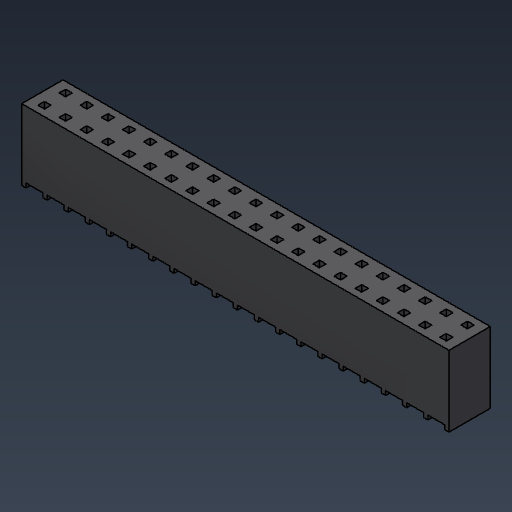
# Autodesk Inventor part: SSW-120-01-F-D_terminal
Saved by Autodesk Inventor 2023.1 (Build 271208000, 208)
## iProperties
Category: PARTsolutions
Company: SAMTEC
Created: 2015-08-09
Part Number: SSW-120-01-F-D_terminal
Catalog Web Link: www.cadenas.de
Description: SSW Series Terminal-SSW Series - (2,54 mm) .100" Surface Mount Terminal & Through-Hole .025" Square Post Socket
Vendor: SAMTEC
Document SubType Name: Modeling
Designer: PARTuser1
Manufacturer: SAMTEC
Mass: 1.8617 g
Surface Area: 24.8346 cm^2
Volume: 1.8617 cm^3
Density: 1 g/cm^3
Material: Allgemein
Appearance: PSOLRGB-175-175-175
PSOL_IDENT_0: {$CADENAS_DATA\23d-libs\samtec\modelling\ssw\parts\ssw_terminal.prj},256 {VTYP=3D},{NB=SSW-120-01-F-
PSOL_IDENT_1: D_terminal},{LINA=SSW-120-01-F-D_terminal},{NN=SSW Series Terminal},{DATE=20.05.2015 07:57:00},{GEOM
PSOL_IDENT_2: DATE=20.05.2015 07:56:00},{VERSION=},{LINEID=10},{LINESUBID=-1},{WBVAR=POS,LS,PLOPT,ROW,TOPT,POLOPT,
PSOL_IDENT_3: NOPT,LLOPT,POPT,KOPT,TROPT}  {NB=SSW-120-01-F-D_terminal},{LINA=SSW-120-01-F-D_terminal},{KT=DUMMY},
PSOL_IDENT_4: {PN=SSW-120-01-F-D},{SERIES=SSW},{POS=20},{POSATOF=20},{LS=01},{LSALG= '01','-01','02','-02','03','-
PSOL_IDENT_5: 03','04','-04','06','-06','21','-21','22','-22','23','-23','24','-24' },{PLOPT=F},{PLOPTALG= 'G','-G
PSOL_IDENT_6: - Gold, 20micro\" Au / 50micro\" Ni Min on Contact, 3micro\" Au / 50micro\" Ni Min on Tail','S','-S
PSOL_IDENT_7: - Selective, 30micro\" Au / 50micro\" Ni Min on Contact, Matte Tin Tail','H','-H - Heavy Gold 30mic
PSOL_IDENT_8: ro\" Au / 50micro\" Ni Min on Contact, 3micro\" Au / 50micro\" Ni Min on Tail' ,'F','-F - Flash Sele
PSOL_IDENT_9: ctive, 3micro\" Au / 50micro\" Ni Min on Contact, Matte Tin Tail','STL','-STL - Selective, 30micro\"
PSOL_IDENT_10: Au / 50micro\" Ni Min on Contact Area, Tin/Lead (90/10 +/-5%) Tail','SM','-SM - Selective, 30micro\
PSOL_IDENT_11: " Au / 50micro\" Ni Min on Contact, Matte Tin Tail','FM','-FM - Flash Selective, 3micro\" Au / 50mic
PSOL_IDENT_12: ro\" Ni Min on Contact, Matte Tin Tail','L','-L - Light Selective, 10micro\" Au / 50micro\" Ni Min o
PSOL_IDENT_13: n Contact Area, Matte Tin Tail','T','-T - Matte Tin Contact and Tail','E','-E - 50micro\" Extra Heav
PSOL_IDENT_14: y Gold in Contact Area, 3micro\" Gold on Tail','TL','-TL - Tin/Lead (90/10 ± 5%) Contact and Tail','
PSOL_IDENT_15: TM','-TM - Matte Tin Contact and Tail' },{ROW=D},{ROWALG= 'S','-S - Single','D','-D - Double','T','-
PSOL_IDENT_16: T - Triple', 'P','-P - Single Notched','Q','-Q - Triple with only Outer 2 Rows Filled' },{TOPT=},{TO
PSOL_IDENT_17: PTALG= '','Straight' },{TOPTPN=},{POLOPT=},{POLOPTALG= '','Not Selected','001','001','002','002','00
PSOL_IDENT_18: 3','003','004','004','005','005','006','006','007','007','008','008','009','009','010','010','011','
PSOL_IDENT_19: 011','012','012','013','013','014','014','015','015','016','016','017','017','018','018','019','019'
PSOL_IDENT_20: ,'020','020','021','021','022','022','023','023','024','024','025','025','026','026','027','027','02
PSOL_IDENT_21: 8','028','029','029','030','030','031','031','032','032','033','033','034','034','035','035','036','
PSOL_IDENT_22: 036','037','037','038','038','039','039','040','040' },{POLOPTMAX=480},{POLOPTMAX2='001','001','002'
PSOL_IDENT_23: ,'002','003','003','004','004','005','005','006','006','007','007','008','008','009','009','010','01
PSOL_IDENT_24: 0','011','011','012','012','013','013','014','014','015','015','016','016','017','017','018','018','
PSOL_IDENT_25: 019','019','020','020','021','021','022','022','023','023','024','024','025','025','026','026','027'
PSOL_IDENT_26: ,'027','028','028','029','029','030','030','031','031','032','032','033','033','034','034','035','03
PSOL_IDENT_27: 5','036','036','037','037','038','038','039','039','040','040'},{POLARIZE='001','001','002','002','0
PSOL_IDENT_28: 03','003','004','004','005','005','006','006','007','007','008','008','009','009','010','010','011','
PSOL_IDENT_29: 011','012','012','013','013','014','014','015','015','016','016','017','017','018','018','019','019'
PSOL_IDENT_30: ,'020','020','021','021','022','022','023','023','024','024','025','025','026','026','027','027','02
PSOL_IDENT_31: 8','028','029','029','030','030','031','031','032','032','033','033','034','034','035','035','036','
PSOL_IDENT_32: 036','037','037','038','038','039','039','040','040','041','041','042','042','043','043','044','044'
PSOL_IDENT_33: ,'045','045','046','046','047','047','048','048','049','049','050','050','051','051','052','052','05
PSOL_IDENT_34: 3','053','054','054','055','055','056','056','057','057','058','058','059','059','060','060','061','
PSOL_IDENT_35: 061','062','062','063','063','064','064','065','065','066','066','067','067','068','068','069','069'
PSOL_IDENT_36: ,'070','070','071','071','072','072','073','073','074','074','075','075','076','076','077','077','07
PSOL_IDENT_37: 8','078','079','079','080','080','081','081','082','082','083','083','084','084','085','085','086','
PSOL_IDENT_38: 086','087','087','088','088','089','089','090','090','091','091','092','092','093','093','094','094'
PSOL_IDENT_39: ,'095','095','096','096','097','097','098','098','099','099','100','100','101','101','102','102','10
PSOL_IDENT_40: 3','103','104','104','105','105','106','106','107','107','108','108','109','109','110','110','111','
PSOL_IDENT_41: 111','112','112','113','113','114','114','115','115','116','116','117','117','118','118','119','119'
PSOL_IDENT_42: ,'120','120','121','121','122','122','123','123','124','124','125','125','126','126','127','127','12
PSOL_IDENT_43: 8','128','129','129','130','130','131','131','132','132','133','133','134','134','135','135','136','
PSOL_IDENT_44: 136','137','137','138','138','139','139','140','140','141','141','142','142','143','143','144','144'
PSOL_IDENT_45: ,'145','145','146','146','147','147','148','148','149','149','150','150'},{POLOPTPN=},{NOPT=},{NOPTA
PSOL_IDENT_46: LG= '','Not Selected','N','-N - Notch' },{NOPTPN=},{LLOPT=},{LLOPTALG= '','Not Selected','LL','-LL -
PSOL_IDENT_47: Locking Lead' },{LLOPTPN=},{POPT=},{POPTALG= '','Not Available' },{POPTPN=},{KOPT=},{KOPTALG= '','N
PSOL_IDENT_48: ot Available' },{KOPTPN=},{TROPT=},{TROPTALG= '','Not Available' },{TROPTPN=},{B=0.104},{C=0.000},{R=
PSOL_IDENT_49: 2.020},{APOPT=0.81250},{CPOPT=0.89750},{SKOPT=0.88200},{OEN=2},{POSX=1.01500},{POSY=0.01500},{POLOPT
PSOL_IDENT_50: ATOF=0},{POLMOVE=2}
NN: SSW Series Terminal
NT: SSW Series - (2,54 mm) .100" Surface Mount Terminal & Through-Hole .025" Square Post Socket
NB: SSW-120-01-F-D_terminal
NBSYN: $PN._terminal
LINA: SSW-120-01-F-D_terminal
SERIES: SSW
POS: -20
LS: -01
PLOPT: -F - Flash Selective, 3micro" Au / 50micro" Ni Min on Contact, Matte Tin Tail
ROW: -D - Double
TOPT: Straight
POLOPT: Not Selected
NOPT: Not Selected
LLOPT: Not Selected
POPT: Not Available
KOPT: Not Available
TROPT: Not Available
SUPPLIER: SAMTEC
ARTICLENO: SSW-120-01-F-D_terminal
BOMINFO: SSW-120-01-F-D_terminal
CREATOR: CADENAS GmbH
Title: SSW-120-01-F-D_terminal
Author: Cadenas PARTsolutions
Comments: SSW Series - (2,54 mm) .100" Surface Mount Terminal & Through-Hole .025" Square Post Socket
Autodesk Inventor part; units mm, degrees
sketch "Sketch_1" plane through (0, 0, 0) normal (0, 1, 0) x (-1, 0, 0)
  line L0 (25.654, -2.4765) -> (25.654, 2.4765)
  line L1 (25.654, 2.4765) -> (-25.654, 2.4765)
  line L2 (-25.654, 2.4765) -> (-25.654, -2.4765)
  line L3 (-25.654, -2.4765) -> (25.654, -2.4765)
  line L4 (-23.7363, 0.8763) -> (-23.7363, 1.6637)
  line L5 (-23.7363, 1.6637) -> (-24.5237, 1.6637)
  line L6 (-24.5237, 1.6637) -> (-24.5237, 0.8763)
  line L7 (-24.5237, 0.8763) -> (-23.7363, 0.8763)
  line L8 (-23.7363, -1.6637) -> (-23.7363, -0.8763)
  line L9 (-23.7363, -0.8763) -> (-24.5237, -0.8763)
  line L10 (-24.5237, -0.8763) -> (-24.5237, -1.6637)
  line L11 (-24.5237, -1.6637) -> (-23.7363, -1.6637)
  line L12 (-21.1963, 0.8763) -> (-21.1963, 1.6637)
  line L13 (-21.1963, 1.6637) -> (-21.9837, 1.6637)
  line L14 (-21.9837, 1.6637) -> (-21.9837, 0.8763)
  line L15 (-21.9837, 0.8763) -> (-21.1963, 0.8763)
  line L16 (-21.1963, -1.6637) -> (-21.1963, -0.8763)
  line L17 (-21.1963, -0.8763) -> (-21.9837, -0.8763)
  line L18 (-21.9837, -0.8763) -> (-21.9837, -1.6637)
  line L19 (-21.9837, -1.6637) -> (-21.1963, -1.6637)
  line L20 (-18.6563, 0.8763) -> (-18.6563, 1.6637)
  line L21 (-18.6563, 1.6637) -> (-19.4437, 1.6637)
  line L22 (-19.4437, 1.6637) -> (-19.4437, 0.8763)
  line L23 (-19.4437, 0.8763) -> (-18.6563, 0.8763)
  line L24 (-18.6563, -1.6637) -> (-18.6563, -0.8763)
  line L25 (-18.6563, -0.8763) -> (-19.4437, -0.8763)
  line L26 (-19.4437, -0.8763) -> (-19.4437, -1.6637)
  line L27 (-19.4437, -1.6637) -> (-18.6563, -1.6637)
  line L28 (-16.1163, 0.8763) -> (-16.1163, 1.6637)
  line L29 (-16.1163, 1.6637) -> (-16.9037, 1.6637)
  line L30 (-16.9037, 1.6637) -> (-16.9037, 0.8763)
  line L31 (-16.9037, 0.8763) -> (-16.1163, 0.8763)
  line L32 (-16.1163, -1.6637) -> (-16.1163, -0.8763)
  line L33 (-16.1163, -0.8763) -> (-16.9037, -0.8763)
  line L34 (-16.9037, -0.8763) -> (-16.9037, -1.6637)
  line L35 (-16.9037, -1.6637) -> (-16.1163, -1.6637)
  line L36 (-13.5763, 0.8763) -> (-13.5763, 1.6637)
  line L37 (-13.5763, 1.6637) -> (-14.3637, 1.6637)
  line L38 (-14.3637, 1.6637) -> (-14.3637, 0.8763)
  line L39 (-14.3637, 0.8763) -> (-13.5763, 0.8763)
  line L40 (-13.5763, -1.6637) -> (-13.5763, -0.8763)
  line L41 (-13.5763, -0.8763) -> (-14.3637, -0.8763)
  line L42 (-14.3637, -0.8763) -> (-14.3637, -1.6637)
  line L43 (-14.3637, -1.6637) -> (-13.5763, -1.6637)
  line L44 (-11.0363, 0.8763) -> (-11.0363, 1.6637)
  line L45 (-11.0363, 1.6637) -> (-11.8237, 1.6637)
  line L46 (-11.8237, 1.6637) -> (-11.8237, 0.8763)
  line L47 (-11.8237, 0.8763) -> (-11.0363, 0.8763)
  line L48 (-11.0363, -1.6637) -> (-11.0363, -0.8763)
  line L49 (-11.0363, -0.8763) -> (-11.8237, -0.8763)
  line L50 (-11.8237, -0.8763) -> (-11.8237, -1.6637)
  line L51 (-11.8237, -1.6637) -> (-11.0363, -1.6637)
  line L52 (-8.4963, 0.8763) -> (-8.4963, 1.6637)
  line L53 (-8.4963, 1.6637) -> (-9.2837, 1.6637)
  line L54 (-9.2837, 1.6637) -> (-9.2837, 0.8763)
  line L55 (-9.2837, 0.8763) -> (-8.4963, 0.8763)
  line L56 (-8.4963, -1.6637) -> (-8.4963, -0.8763)
  line L57 (-8.4963, -0.8763) -> (-9.2837, -0.8763)
  line L58 (-9.2837, -0.8763) -> (-9.2837, -1.6637)
  line L59 (-9.2837, -1.6637) -> (-8.4963, -1.6637)
  line L60 (-5.9563, 0.8763) -> (-5.9563, 1.6637)
  line L61 (-5.9563, 1.6637) -> (-6.7437, 1.6637)
  line L62 (-6.7437, 1.6637) -> (-6.7437, 0.8763)
  line L63 (-6.7437, 0.8763) -> (-5.9563, 0.8763)
  line L64 (-5.9563, -1.6637) -> (-5.9563, -0.8763)
  line L65 (-5.9563, -0.8763) -> (-6.7437, -0.8763)
  line L66 (-6.7437, -0.8763) -> (-6.7437, -1.6637)
  line L67 (-6.7437, -1.6637) -> (-5.9563, -1.6637)
  line L68 (-3.4163, 0.8763) -> (-3.4163, 1.6637)
  line L69 (-3.4163, 1.6637) -> (-4.2037, 1.6637)
  line L70 (-4.2037, 1.6637) -> (-4.2037, 0.8763)
  line L71 (-4.2037, 0.8763) -> (-3.4163, 0.8763)
  line L72 (-3.4163, -1.6637) -> (-3.4163, -0.8763)
  line L73 (-3.4163, -0.8763) -> (-4.2037, -0.8763)
  line L74 (-4.2037, -0.8763) -> (-4.2037, -1.6637)
  line L75 (-4.2037, -1.6637) -> (-3.4163, -1.6637)
  line L76 (-0.8763, 0.8763) -> (-0.8763, 1.6637)
  line L77 (-0.8763, 1.6637) -> (-1.6637, 1.6637)
  line L78 (-1.6637, 1.6637) -> (-1.6637, 0.8763)
  line L79 (-1.6637, 0.8763) -> (-0.8763, 0.8763)
  line L80 (-0.8763, -1.6637) -> (-0.8763, -0.8763)
  line L81 (-0.8763, -0.8763) -> (-1.6637, -0.8763)
  line L82 (-1.6637, -0.8763) -> (-1.6637, -1.6637)
  line L83 (-1.6637, -1.6637) -> (-0.8763, -1.6637)
  line L84 (1.6637, 0.8763) -> (1.6637, 1.6637)
  line L85 (1.6637, 1.6637) -> (0.8763, 1.6637)
  line L86 (0.8763, 1.6637) -> (0.8763, 0.8763)
  line L87 (0.8763, 0.8763) -> (1.6637, 0.8763)
  line L88 (1.6637, -1.6637) -> (1.6637, -0.8763)
  line L89 (1.6637, -0.8763) -> (0.8763, -0.8763)
  line L90 (0.8763, -0.8763) -> (0.8763, -1.6637)
  line L91 (0.8763, -1.6637) -> (1.6637, -1.6637)
  line L92 (4.2037, 0.8763) -> (4.2037, 1.6637)
  line L93 (4.2037, 1.6637) -> (3.4163, 1.6637)
  line L94 (3.4163, 1.6637) -> (3.4163, 0.8763)
  line L95 (3.4163, 0.8763) -> (4.2037, 0.8763)
  line L96 (4.2037, -1.6637) -> (4.2037, -0.8763)
  line L97 (4.2037, -0.8763) -> (3.4163, -0.8763)
  line L98 (3.4163, -0.8763) -> (3.4163, -1.6637)
  line L99 (3.4163, -1.6637) -> (4.2037, -1.6637)
  line L100 (6.7437, 0.8763) -> (6.7437, 1.6637)
  line L101 (6.7437, 1.6637) -> (5.9563, 1.6637)
  line L102 (5.9563, 1.6637) -> (5.9563, 0.8763)
  line L103 (5.9563, 0.8763) -> (6.7437, 0.8763)
  line L104 (6.7437, -1.6637) -> (6.7437, -0.8763)
  line L105 (6.7437, -0.8763) -> (5.9563, -0.8763)
  line L106 (5.9563, -0.8763) -> (5.9563, -1.6637)
  line L107 (5.9563, -1.6637) -> (6.7437, -1.6637)
  line L108 (9.2837, 0.8763) -> (9.2837, 1.6637)
  line L109 (9.2837, 1.6637) -> (8.4963, 1.6637)
  line L110 (8.4963, 1.6637) -> (8.4963, 0.8763)
  line L111 (8.4963, 0.8763) -> (9.2837, 0.8763)
  line L112 (9.2837, -1.6637) -> (9.2837, -0.8763)
  line L113 (9.2837, -0.8763) -> (8.4963, -0.8763)
  line L114 (8.4963, -0.8763) -> (8.4963, -1.6637)
  line L115 (8.4963, -1.6637) -> (9.2837, -1.6637)
  line L116 (11.8237, 0.8763) -> (11.8237, 1.6637)
  line L117 (11.8237, 1.6637) -> (11.0363, 1.6637)
  line L118 (11.0363, 1.6637) -> (11.0363, 0.8763)
  line L119 (11.0363, 0.8763) -> (11.8237, 0.8763)
  line L120 (11.8237, -1.6637) -> (11.8237, -0.8763)
  line L121 (11.8237, -0.8763) -> (11.0363, -0.8763)
  line L122 (11.0363, -0.8763) -> (11.0363, -1.6637)
  line L123 (11.0363, -1.6637) -> (11.8237, -1.6637)
  line L124 (14.3637, 0.8763) -> (14.3637, 1.6637)
  line L125 (14.3637, 1.6637) -> (13.5763, 1.6637)
  line L126 (13.5763, 1.6637) -> (13.5763, 0.8763)
  line L127 (13.5763, 0.8763) -> (14.3637, 0.8763)
  line L128 (14.3637, -1.6637) -> (14.3637, -0.8763)
  line L129 (14.3637, -0.8763) -> (13.5763, -0.8763)
  line L130 (13.5763, -0.8763) -> (13.5763, -1.6637)
  line L131 (13.5763, -1.6637) -> (14.3637, -1.6637)
  line L132 (16.9037, 0.8763) -> (16.9037, 1.6637)
  line L133 (16.9037, 1.6637) -> (16.1163, 1.6637)
  line L134 (16.1163, 1.6637) -> (16.1163, 0.8763)
  line L135 (16.1163, 0.8763) -> (16.9037, 0.8763)
  line L136 (16.9037, -1.6637) -> (16.9037, -0.8763)
  line L137 (16.9037, -0.8763) -> (16.1163, -0.8763)
  line L138 (16.1163, -0.8763) -> (16.1163, -1.6637)
  line L139 (16.1163, -1.6637) -> (16.9037, -1.6637)
  line L140 (19.4437, 0.8763) -> (19.4437, 1.6637)
  line L141 (19.4437, 1.6637) -> (18.6563, 1.6637)
  line L142 (18.6563, 1.6637) -> (18.6563, 0.8763)
  line L143 (18.6563, 0.8763) -> (19.4437, 0.8763)
  line L144 (19.4437, -1.6637) -> (19.4437, -0.8763)
  line L145 (19.4437, -0.8763) -> (18.6563, -0.8763)
  line L146 (18.6563, -0.8763) -> (18.6563, -1.6637)
  line L147 (18.6563, -1.6637) -> (19.4437, -1.6637)
  line L148 (21.9837, 0.8763) -> (21.9837, 1.6637)
  line L149 (21.9837, 1.6637) -> (21.1963, 1.6637)
  line L150 (21.1963, 1.6637) -> (21.1963, 0.8763)
  line L151 (21.1963, 0.8763) -> (21.9837, 0.8763)
  line L152 (21.9837, -1.6637) -> (21.9837, -0.8763)
  line L153 (21.9837, -0.8763) -> (21.1963, -0.8763)
  line L154 (21.1963, -0.8763) -> (21.1963, -1.6637)
  line L155 (21.1963, -1.6637) -> (21.9837, -1.6637)
  line L156 (24.5237, 0.8763) -> (24.5237, 1.6637)
  line L157 (24.5237, 1.6637) -> (23.7363, 1.6637)
  line L158 (23.7363, 1.6637) -> (23.7363, 0.8763)
  line L159 (23.7363, 0.8763) -> (24.5237, 0.8763)
  line L160 (24.5237, -1.6637) -> (24.5237, -0.8763)
  line L161 (24.5237, -0.8763) -> (23.7363, -0.8763)
  line L162 (23.7363, -0.8763) -> (23.7363, -1.6637)
  line L163 (23.7363, -1.6637) -> (24.5237, -1.6637)
  constraints: 328 end point
extrude "Extrusion1" add sketch "Sketch_1" along normal blind 8.509
sketch "Sketch_6" plane through (0, 0, 0) normal (0, 0, 1) x (1, 0, 0)
  line L0 (-25.146, -2.032) -> (25.146, -2.032)
  line L1 (25.146, -2.032) -> (25.146, 0.508)
  line L2 (25.146, 0.508) -> (23.114, 0.508)
  line L3 (23.114, 0.508) -> (23.114, -1.27)
  line L4 (23.114, -1.27) -> (22.606, -1.27)
  line L5 (22.606, -1.27) -> (22.606, 0.508)
  line L6 (22.606, 0.508) -> (20.574, 0.508)
  line L7 (20.574, 0.508) -> (20.574, -1.27)
  line L8 (20.574, -1.27) -> (20.066, -1.27)
  line L9 (20.066, -1.27) -> (20.066, 0.508)
  line L10 (20.066, 0.508) -> (18.034, 0.508)
  line L11 (18.034, 0.508) -> (18.034, -1.27)
  line L12 (18.034, -1.27) -> (17.526, -1.27)
  line L13 (17.526, -1.27) -> (17.526, 0.508)
  line L14 (17.526, 0.508) -> (15.494, 0.508)
  line L15 (15.494, 0.508) -> (15.494, -1.27)
  line L16 (15.494, -1.27) -> (14.986, -1.27)
  line L17 (14.986, -1.27) -> (14.986, 0.508)
  line L18 (14.986, 0.508) -> (12.954, 0.508)
  line L19 (12.954, 0.508) -> (12.954, -1.27)
  line L20 (12.954, -1.27) -> (12.446, -1.27)
  line L21 (12.446, -1.27) -> (12.446, 0.508)
  line L22 (12.446, 0.508) -> (10.414, 0.508)
  line L23 (10.414, 0.508) -> (10.414, -1.27)
  line L24 (10.414, -1.27) -> (9.906, -1.27)
  line L25 (9.906, -1.27) -> (9.906, 0.508)
  line L26 (9.906, 0.508) -> (7.874, 0.508)
  line L27 (7.874, 0.508) -> (7.874, -1.27)
  line L28 (7.874, -1.27) -> (7.366, -1.27)
  line L29 (7.366, -1.27) -> (7.366, 0.508)
  line L30 (7.366, 0.508) -> (5.334, 0.508)
  line L31 (5.334, 0.508) -> (5.334, -1.27)
  line L32 (5.334, -1.27) -> (4.826, -1.27)
  line L33 (4.826, -1.27) -> (4.826, 0.508)
  line L34 (4.826, 0.508) -> (2.794, 0.508)
  line L35 (2.794, 0.508) -> (2.794, -1.27)
  line L36 (2.794, -1.27) -> (2.286, -1.27)
  line L37 (2.286, -1.27) -> (2.286, 0.508)
  line L38 (2.286, 0.508) -> (0.254, 0.508)
  line L39 (0.254, 0.508) -> (0.254, -1.27)
  line L40 (0.254, -1.27) -> (-0.254, -1.27)
  line L41 (-0.254, -1.27) -> (-0.254, 0.508)
  line L42 (-0.254, 0.508) -> (-2.286, 0.508)
  line L43 (-2.286, 0.508) -> (-2.286, -1.27)
  line L44 (-2.286, -1.27) -> (-2.794, -1.27)
  line L45 (-2.794, -1.27) -> (-2.794, 0.508)
  line L46 (-2.794, 0.508) -> (-4.826, 0.508)
  line L47 (-4.826, 0.508) -> (-4.826, -1.27)
  line L48 (-4.826, -1.27) -> (-5.334, -1.27)
  line L49 (-5.334, -1.27) -> (-5.334, 0.508)
  line L50 (-5.334, 0.508) -> (-7.366, 0.508)
  line L51 (-7.366, 0.508) -> (-7.366, -1.27)
  line L52 (-7.366, -1.27) -> (-7.874, -1.27)
  line L53 (-7.874, -1.27) -> (-7.874, 0.508)
  line L54 (-7.874, 0.508) -> (-9.906, 0.508)
  line L55 (-9.906, 0.508) -> (-9.906, -1.27)
  line L56 (-9.906, -1.27) -> (-10.414, -1.27)
  line L57 (-10.414, -1.27) -> (-10.414, 0.508)
  line L58 (-10.414, 0.508) -> (-12.446, 0.508)
  line L59 (-12.446, 0.508) -> (-12.446, -1.27)
  line L60 (-12.446, -1.27) -> (-12.954, -1.27)
  line L61 (-12.954, -1.27) -> (-12.954, 0.508)
  line L62 (-12.954, 0.508) -> (-14.986, 0.508)
  line L63 (-14.986, 0.508) -> (-14.986, -1.27)
  line L64 (-14.986, -1.27) -> (-15.494, -1.27)
  line L65 (-15.494, -1.27) -> (-15.494, 0.508)
  line L66 (-15.494, 0.508) -> (-17.526, 0.508)
  line L67 (-17.526, 0.508) -> (-17.526, -1.27)
  line L68 (-17.526, -1.27) -> (-18.034, -1.27)
  line L69 (-18.034, -1.27) -> (-18.034, 0.508)
  line L70 (-18.034, 0.508) -> (-20.066, 0.508)
  line L71 (-20.066, 0.508) -> (-20.066, -1.27)
  line L72 (-20.066, -1.27) -> (-20.574, -1.27)
  line L73 (-20.574, -1.27) -> (-20.574, 0.508)
  line L74 (-20.574, 0.508) -> (-22.606, 0.508)
  line L75 (-22.606, 0.508) -> (-22.606, -1.27)
  line L76 (-22.606, -1.27) -> (-23.114, -1.27)
  line L77 (-23.114, -1.27) -> (-23.114, 0.508)
  line L78 (-23.114, 0.508) -> (-25.146, 0.508)
  line L79 (-25.146, 0.508) -> (-25.146, -2.032)
  constraints: 160 end point
extrude "Extrusion2" cut sketch "Sketch_6" along normal mid plane 10.16
ref_plane "pin_XY" through (0, 0, 0) normal (0, 1, 0) x (1, 0, 0)
ref_plane "pin_YZ" through (0, 0, 0) normal (1, 0, 0) x (0, 0, -1)
ref_plane "pin_ZX" through (0, 0, 0) normal (0, 0, -1) x (0, 1, 0)
ref_plane "terminal_XY" through (0, 0, 0) normal (0, -1, 0) x (1, 0, 0)
ref_plane "terminal_YZ" through (0, 0, 0) normal (1, 0, 0) x (0, 0, 1)
ref_plane "terminal_ZX" through (0, 0, 0) normal (0, 0, 1) x (0, -1, 0)
body "Solid1"
